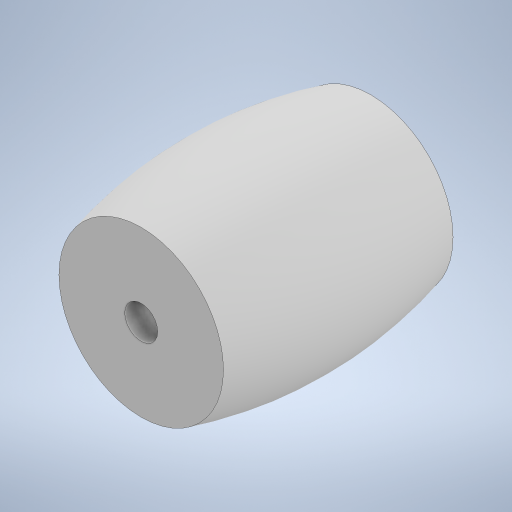
# Autodesk Inventor part: OmnorollerV4
Saved by Autodesk Inventor 2024 (Build 280153000, 153)
## iProperties
Created: 2023-11-15
Part Number: OmnorollerV4
Material: Generic
Document SubType Name: Modeling
Designer: felip
Density: 1 g/cm^3
Appearance: Default
Author: felip
Autodesk Inventor part; units mm, degrees
ref_plane "YZ Plane" through (0, 0, 0) normal (1, 0, 0) x (0, 1, 0)
ref_plane "XZ Plane" through (0, 0, 0) normal (0, 1, 0) x (-1, 0, 0)
ref_plane "XY Plane" through (0, 0, 0) normal (0, 0, 1) x (1, 0, 0)
sketch "Sketch1" plane through (0, 0, 0) normal (0, 1, 0) x (-1, 0, 0)
  arc A0 (29.4321, -8) -> (29.4321, 8) centre (0, 0) ccw
  line L0 (30.5, 0) -> (23.7, 0)
  line L1 (23.7, 0) -> (23.7, -8)
  line L2 (23.7, 0) -> (23.7, 8)
  line L3 (23.7, 8) -> (29.4321, 8)
  line L4 (23.7, -8) -> (29.4321, -8)
  dimension "d3" = 61
  dimension "d4" = 6.8
  dimension "d5" = 8
  dimension "d6" = 8
  constraints: 10 end point, 3 point on circle, 2 horizontal, 1 centre point, 1 coincident, 1 parallel, 1 perpendicular, 1 vertical
  measures "d3" diameter of A0
  measures "d4" distance of L0.start L0.end
  measures "d5" distance of L0.end L1.end
  measures "d6" distance of L0.end L2.end
revolve "Revolution1" add sketch "Sketch1" angle 360 about axis through (-23.7, 0, 0) along (0, 0, 1)
sketch "Sketch2" plane through (-23.7, 0, 8) normal (0, 0, 1) x (1, 0, 0)
  circle A0 centre (0, 0) radius 1.15
  point P0 (23.7, 0)
  dimension "d8" = 2.3
  constraints: 1 centre point
  measures "d8" diameter of A0
extrude "Extrusion1" cut sketch "Sketch2" against normal blind 30
body "Solid1"
